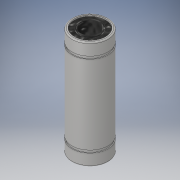
# Autodesk Inventor part: lm8luu
Saved by Autodesk Inventor 2018 (Build 220112000, 112)
## iProperties
Created: 2017-11-18
Part Number: lm8luu
Material: Edelstahl, 440C
Document SubType Name: Modeling
Designer: Till
Density: 7.75 g/cm^3
Appearance: Poliert - Silber
Author: Till
Autodesk Inventor part; units mm, degrees
ref_plane "YZ Plane" through (0, 0, 0) normal (1, 0, 0) x (0, 1, 0)
ref_plane "XZ Plane" through (0, 0, 0) normal (0, 1, 0) x (-1, 0, 0)
ref_plane "XY Plane" through (0, 0, 0) normal (0, 0, 1) x (1, 0, 0)
sketch "Skizze2" plane through (0, 0, 0) normal (1, 0, 0) x (0, 1, 0)
  line L0 (4.5, 0) -> (4.5, 0.5)
  line L1 (4.5, 0) -> (5, 0) construction
  line L2 (4.5, 0.5) -> (6.5, 0.5)
  line L3 (6.5, 0.5) -> (6.5, 0)
  line L4 (6.5, 0) -> (7, 0)
  line L5 (4.5, 0) -> (4, 0)
  line L6 (4, 0) -> (4, 45)
  line L7 (4, 45) -> (4.5, 45)
  line L8 (4.5, 45) -> (4.5, 44.5)
  line L9 (4.5, 44.5) -> (6.5, 44.5)
  line L10 (6.5, 44.5) -> (6.5, 45)
  line L11 (6.5, 45) -> (7, 45)
  arc A0 (7.5, 44.5) -> (7, 45) centre (7, 44.5) ccw
  arc A1 (7, 0) -> (7.5, 0.5) centre (7, 0.5) ccw
  line L12 (0, -9.145) -> (0, 54.145) projected
  line L13 (7.5, 0.5) -> (7.5, 5)
  line L14 (7.5, 5) -> (7.15, 5)
  line L15 (7.15, 5) -> (7.15, 6.1)
  line L16 (7.15, 6.1) -> (7.5, 6.1)
  line L17 (7.5, 6.1) -> (7.5, 38.9)
  line L18 (7.5, 38.9) -> (7.15, 38.9)
  line L19 (7.15, 38.9) -> (7.15, 40)
  line L20 (7.15, 40) -> (7.5, 40)
  line L21 (7.5, 40) -> (7.5, 44.5)
  point P0 (0, 0)
  point P1 (7.5, 0)
  point P2 (7.5, 45)
  dimension "d1" = 0.5
  dimension "d2" = 90
  dimension "d4" = 1
  dimension "d7" = 0.5
  dimension "d8" = 45
  dimension "d10" = 0.5
  dimension "d12" = 0.5
  dimension "d14" = 4
  dimension "d16" = 1
  dimension "d17" = 0.5
  dimension "d18" = 0
  dimension "d19" = 0.5
  dimension "d24" = 1.1
  dimension "d25" = 1.1
  dimension "d26" = 0.35
  dimension "d27" = 0.35
  dimension "d29" = 2
  dimension "d30" = 2
  dimension "d31" = 5
  dimension "d33" = 1
  dimension "d34" = 0.5
  dimension "d35" = 0.5
  dimension "d36" = 0.5
  dimension "d37" = 0
  dimension "d38" = 35
  constraints: 42 end point, 17 perpendicular, 4 point on circle, 4 point on line, 2 centre point, 2 horizontal, 2 tangent, 1 equal radius, 1 vertical
  measures "d1" distance of L0.start L0.end
  measures "d2" angle of L1 L0
  measures "d4" distance of L3.end point (7.5, 0)
  measures "d7" distance of L0.start L5.end
  measures "d8" distance of L5.end L6.end
  measures "d10" distance of L6.end L7.end
  measures "d12" distance of L7.end L8.end
  measures "d14" distance from line of point (0, 0) L6
  measures "d16" distance of L10.end point (7.5, 45)
  measures "d17" distance of L9.end L10.end
  measures "d18" distance from line of point (0, 0) L5
  measures "d19" radius of A0
  measures "d24" distance of L18.end L19.end
  measures "d25" distance of L14.end L15.end
  measures "d26" distance of L13.end L14.end
  measures "d27" distance of L17.end L18.end
  measures "d29" distance between parallel lines of L8 L10
  measures "d30" distance of L0.end L2.end
  measures "d31" distance between parallel lines of L14 L4
  measures "d33" distance of L9.end L21.end
  measures "d34" distance of L9.end A0.centre
  measures "d35" distance of L2.end A1.centre
  measures "d36" distance of L2.end L3.end
  measures "d37" distance from line of L2 L13.start
  measures "d38" distance between parallel lines of L14 L20
revolve "Umdrehung1" add sketch "Skizze2" angle 360 about axis through (0, 0, -10) along (0, 0, 1)
